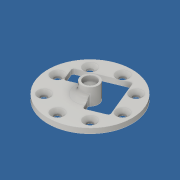
# Autodesk Inventor part: WristMagnetMount
Saved by Autodesk Inventor 2016 (Build 200138000, 138)
## iProperties
Created: 2016-03-29
Part Number: WristMagnetMount
Material: ABS-Kunststoff
Document SubType Name: Modeling
Designer: 4ndreas
Density: 1.06 g/cm^3
Appearance: Glatt - weiß
Mass: 2.46864 g
Surface Area: 26.623 cm^2
Volume: 2.3289 cm^3
Author: 4ndreas
Autodesk Inventor part; units mm, degrees
ref_plane "YZ Plane" through (0, 0, 0) normal (1, 0, 0) x (0, 1, 0)
ref_plane "XZ Plane" through (0, 0, 0) normal (0, 1, 0) x (-1, 0, 0)
ref_plane "XY Plane" through (0, 0, 0) normal (0, 0, 1) x (1, 0, 0)
sketch "Skizze1" plane through (0, 0, 0) normal (0, 0, 1) x (1, 0, 0)
  line L0 (4.368, -7.9322) -> (-3.477, 11.0073)
  line L1 (5.7618, 14.8341) -> (13.6068, -4.1054)
  line L2 (13.6068, -4.1054) -> (4.368, -7.9322)
  circle A0 centre (-10.9602, 10.9602) radius 1.5
  circle A1 centre (10.9602, -10.9602) radius 1.5
  circle A2 centre (15.5, 0) radius 1.5
  circle A3 centre (0, 15.5) radius 1.5
  circle A4 centre (10.9602, 10.9602) radius 1.5
  circle A5 centre (0, -15.5) radius 1.5
  circle A6 centre (0, 0) radius 17.5
  line L3 (-3.477, 11.0073) -> (5.7618, 14.8341)
  point P0 (0, 0)
  constraints: 8 end point, 7 centre point
extrude "Extrusion1" add sketch "Skizze1" along normal blind 3.5
sketch "Skizze2" plane through (0, 0, 3.5) normal (0, 0, 1) x (1, 0, 0)
  circle A0 centre (0, 0) radius 20 projected
  line L0 (5.7618, 14.8341) -> (13.6068, -4.1054) projected
  line L1 (13.6068, -4.1054) -> (4.368, -7.9322) projected
  line L2 (4.368, -7.9322) -> (-3.477, 11.0073) projected
  circle A1 centre (0, -15.5) radius 1.5 projected
  circle A2 centre (10.9602, 10.9602) radius 1.5 projected
  circle A3 centre (0, 15.5) radius 1.5 projected
  circle A4 centre (15.5, 0) radius 1.5 projected
  circle A5 centre (10.9602, -10.9602) radius 1.5 projected
  circle A6 centre (-10.9602, 10.9602) radius 1.5 projected
  circle A7 centre (0, 0) radius 17.5 projected
  line L3 (-3.477, 11.0073) -> (5.7618, 14.8341) projected
  point P0 (0, 0)
extrude "Extrusion2" add sketch "Skizze2" along normal blind 2.4 contours A0 | A7
sketch "Skizze3" plane through (0, 0, 5.9) normal (0, 0, 1) x (1, 0, 0)
  circle A0 centre (0, 0) radius 4
  circle A1 centre (0, 0) radius 3
  point P0 (0, 0)
  dimension "d4" = 8
  dimension "d5" = 6
  constraints: 2 centre point, 2 coincident
  measures "d4" diameter of A0
  measures "d5" diameter of A1
extrude "Extrusion3" add sketch "Skizze3" against normal up to surface (5.9 mm away) contours A0 | A1
extrude "Extrusion4" cut sketch "Skizze3" against normal blind 2.5 contours A1
fillet "Rundung1" [suppressed]
sketch "Skizze4" plane through (0, 0, 5.9) normal (0, 0, 1) x (1, 0, 0)
  arc A0 (3.1481, -7.6003) -> (3.7791, -7.4419) centre (2.9832, -5.6071) ccw
  line L0 (3.1481, -7.6003) -> (2.4615, -5.9426)
  circle A1 centre (-10.9602, 10.9602) radius 1.5
  circle A2 centre (10.9602, -10.9602) radius 1.5
  circle A3 centre (15.5, 0) radius 1.5
  circle A4 centre (0, 15.5) radius 1.5
  circle A5 centre (10.9602, 10.9602) radius 4.0538
  circle A6 centre (0, -15.5) radius 1.5
  line L1 (7.6537, -18.4776) -> (-7.6537, 18.4776)
  line L2 (3.1481, -7.6003) -> (2.4615, -5.9426)
  circle A7 centre (0, 0) radius 3 projected
  line L3 (-0.5582, 3.9609) -> (-3.477, 11.0073) projected
  line L4 (-3.477, 11.0073) -> (5.7618, 14.8341) projected
  line L5 (5.7618, 14.8341) -> (13.6068, -4.1054) projected
  line L6 (13.6068, -4.1054) -> (4.368, -7.9322) projected
  line L7 (4.368, -7.9322) -> (2.406, -3.1955) projected
  arc A8 (2.406, -3.1955) -> (-0.5582, 3.9609) centre (0, 0) ccw projected
  circle A9 centre (-10.9602, 10.9602) radius 1.5 projected
  circle A10 centre (10.9602, -10.9602) radius 1.5 projected
  circle A11 centre (15.5, 0) radius 1.5 projected
  circle A12 centre (0, 15.5) radius 1.5 projected
  circle A13 centre (10.9602, 10.9602) radius 1.5 projected
  circle A14 centre (0, -15.5) radius 1.5 projected
  circle A15 centre (0, 0) radius 20 projected
  circle A16 centre (0, 0) radius 20 projected
  line L8 (10.9602, 10.9602) -> (15.5, 0) construction
  point P0 (0, 0)
  point P1 (0, 0)
  point P2 (-10.9602, -10.9602)
  point P3 (-15.5, 0)
  constraints: 8 end point, 7 centre point, 6 coincident, 3 midpoint, 2 point on circle, 2 symmetric about line, 1 collinear, 1 parallel, 4 other
hole "Bohrung1" at (-10.9602, -10.9602, 5.9) at (0, -15.5, 5.9) at (10.9602, -10.9602, 5.9) at (15.5, 0, 5.9) at (10.9602, 10.9602, 5.9) at (0, 15.5, 5.9) at (-10.9602, 10.9602, 5.9) at (-15.5, 0, 5.9) direction (0, 0, -1) diameter 3 end through all countersink diameter 6 countersink angle 90
sketch "Skizze6" plane through (0, 0, 5.9) normal (0, 0, 1) x (1, 0, 0)
  circle A0 centre (0, 0) radius 20 projected
  arc A1 (2.0245, 13.2861) -> (0.1339, 12.503) centre (0, 15.5) ccw projected
  line L0 (2.0245, 13.2861) -> (5.7618, 14.8341) projected
  line L1 (5.7618, 14.8341) -> (13.6068, -4.1054) projected
  line L2 (13.6068, -4.1054) -> (4.368, -7.9322) projected
  line L3 (4.368, -7.9322) -> (2.406, -3.1955) projected
  arc A2 (2.406, -3.1955) -> (-0.5582, 3.9609) centre (0, 0) ccw projected
  circle A3 centre (0, 0) radius 3 projected
  circle A4 centre (-15.5, 0) radius 3 projected
  circle A5 centre (15.5, 0) radius 3 projected
  circle A6 centre (0, -15.5) radius 3 projected
  circle A7 centre (-10.9602, -10.9602) radius 3 projected
  circle A8 centre (10.9602, -10.9602) radius 3 projected
  circle A9 centre (10.9602, 10.9602) radius 3 projected
  circle A10 centre (-10.9602, 10.9602) radius 3 projected
  line L4 (-3.477, 11.0073) -> (-0.6069, 4.0782)
  line L5 (-0.6069, 4.0782) -> (-11.9892, -0.6365)
  line L6 (-11.9892, -0.6365) -> (-14.8593, 6.2926)
  line L7 (-14.8593, 6.2926) -> (-3.477, 11.0073)
  circle A11 centre (-15.5, 0) radius 3 projected
  line L8 (-3.477, 11.0073) -> (5.7618, 14.8341) projected
  circle A12 centre (0, 0) radius 4 construction
  arc A13 (-0.5582, 3.9609) -> (-1.5307, 3.6955) centre (0, 0) ccw
  line L9 (-11.9892, -0.6365) -> (-11.9892, -0.6365)
  line L10 (-11.9892, -0.6365) -> (-1.5307, 3.6955)
  line L11 (-0.5582, 3.9609) -> (-3.477, 11.0073) projected
  line L12 (-0.6069, 4.0782) -> (-0.5582, 3.9609)
  line L13 (-3.477, 11.0073) -> (0.1339, 12.503) projected
  line L14 (-0.5582, 3.9609) -> (-3.477, 11.0073) projected
  point P0 (0, 0)
  point P1 (-0.6069, 4.0782)
  constraints: 14 end point, 4 collinear, 2 coincident, 2 parallel, 2 perpendicular, 2 point on circle, 2 point on line, 1 centre point, 1 tangent, 4 other
extrude "Extrusion5" cut sketch "Skizze6" against normal through all contours L4 L5 L6 L7 A10 | L11 A13 L5 | A10 L7 picked at (-9.9675, 8.2612)
fillet "Rundung2" radius 1 6 edges at (4.368, -7.9322, 2.95) (13.6068, -4.1054, 2.95) (5.7618, 14.8341, 2.95) (-14.8593, 6.2926, 2.95) (-11.9892, -0.6365, 2.95) (2.406, -3.1955, 2.95)
sketch "Skizze7" plane through (0, 0, 5.9) normal (0, 0, 1) x (1, 0, 0)
  circle A0 centre (0, 0) radius 3 projected
  circle A1 centre (10.9602, 10.9602) radius 3 projected
  circle A2 centre (10.9602, -10.9602) radius 3 projected
  circle A3 centre (-10.9602, -10.9602) radius 3 projected
  circle A4 centre (0, -15.5) radius 3 projected
  circle A5 centre (15.5, 0) radius 3 projected
  line L0 (-8.9357, 8.7462) -> (0.1339, 12.503) projected
  arc A6 (2.0245, 13.2861) -> (0.1339, 12.503) centre (0, 15.5) ccw projected
  arc A7 (6.1445, 13.9103) -> (4.8379, 14.4514) centre (5.2206, 13.5276) ccw projected
  line L1 (6.1445, 13.9103) -> (13.2241, -3.1815) projected
  arc A8 (12.6829, -4.4881) -> (13.2241, -3.1815) centre (12.3003, -3.5642) ccw projected
  line L2 (12.6829, -4.4881) -> (5.2919, -7.5495) projected
  arc A9 (3.9853, -7.0084) -> (5.2919, -7.5495) centre (4.9092, -6.6257) ccw projected
  line L3 (3.9853, -7.0084) -> (2.6776, -3.8511) projected
  arc A10 (2.8811, -2.7747) -> (2.6776, -3.8511) centre (3.6014, -3.4684) ccw projected
  arc A11 (2.8811, -2.7747) -> (-1.5307, 3.6955) centre (0, 0) ccw projected
  line L4 (-1.5307, 3.6955) -> (-11.0653, -0.2538) projected
  arc A12 (-12.3719, 0.2874) -> (-11.0653, -0.2538) centre (-11.448, 0.6701) ccw projected
  line L5 (-12.3719, 0.2874) -> (-12.7284, 1.1481) projected
  circle A13 centre (-15.5, 0) radius 3 projected
  line L6 (-12.7284, 1.1481) -> (-14.4766, 5.3687) projected
  arc A14 (-13.9354, 6.6753) -> (-14.4766, 5.3687) centre (-13.5527, 5.7514) ccw projected
  arc A15 (-8.9357, 8.7462) -> (-10.8262, 7.9631) centre (-10.9602, 10.9602) ccw projected
  circle A16 centre (0, 0) radius 3 projected
  circle A17 centre (0, 0) radius 20 projected
  circle A18 centre (0, 0) radius 4
  line L7 (2.0245, 13.2861) -> (4.8379, 14.4514) projected
  line L8 (-13.9354, 6.6753) -> (-10.8262, 7.9631) projected
  point P0 (0, 0)
  constraints: 2 concentric, 1 centre point, 1 other
extrude "Extrusion6" add sketch "Skizze7" along normal blind 5.5 contours A11 A18
sketch "Skizze8" plane through (0, 0, 3.4) normal (0, 0, 1) x (1, 0, 0)
  circle A0 centre (0, 0) radius 3 projected
  point P0 (0, 0)
extrude "Extrusion7" add sketch "Skizze8" along normal blind 5.5
sketch "Skizze9" plane through (0, 0, 0) normal (0, 0, -1) x (-1, 0, 0)
  line L0 (-4.8379, 14.4514) -> (13.9354, 6.6753) projected
  arc A0 (14.4766, 5.3687) -> (13.9354, 6.6753) centre (13.5527, 5.7514) ccw projected
  line L1 (14.4766, 5.3687) -> (12.3719, 0.2874) projected
  arc A1 (11.0653, -0.2538) -> (12.3719, 0.2874) centre (11.448, 0.6701) ccw projected
  line L2 (11.0653, -0.2538) -> (1.5307, 3.6955) projected
  arc A2 (1.5307, 3.6955) -> (-2.8811, -2.7747) centre (0, 0) ccw projected
  arc A3 (-2.6776, -3.8511) -> (-2.8811, -2.7747) centre (-3.6014, -3.4684) ccw projected
  line L3 (-2.6776, -3.8511) -> (-3.9853, -7.0084) projected
  arc A4 (-5.2919, -7.5495) -> (-3.9853, -7.0084) centre (-4.9092, -6.6257) ccw projected
  line L4 (-5.2919, -7.5495) -> (-12.6829, -4.4881) projected
  arc A5 (-13.2241, -3.1815) -> (-12.6829, -4.4881) centre (-12.3003, -3.5642) ccw projected
  line L5 (-13.2241, -3.1815) -> (-6.1445, 13.9103) projected
  arc A6 (-4.8379, 14.4514) -> (-6.1445, 13.9103) centre (-5.2206, 13.5276) ccw projected
  circle A7 centre (0, -15.5) radius 1.5 projected
  circle A8 centre (-10.9602, 10.9602) radius 1.5 projected
  circle A9 centre (0, 15.5) radius 1.5 projected
  circle A10 centre (-15.5, 0) radius 1.5 projected
  circle A11 centre (-10.9602, -10.9602) radius 1.5 projected
  circle A12 centre (10.9602, 10.9602) radius 1.5 projected
  circle A13 centre (0, 0) radius 17.5 projected
  circle A14 centre (15.5, 0) radius 1.5 projected
  circle A15 centre (10.9602, -10.9602) radius 1.5 projected
  point P0 (0, 0)
extrude "Extrusion8" cut sketch "Skizze9" against normal up to surface (3.5 mm away)
fillet "Rundung3" radius 3 1 edges at (-3.3048, -2.2535, 5.9)
